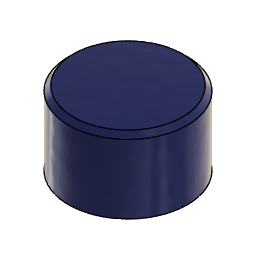
MacropadV2.0 v51 (Autodesk Fusion 360 archive; units mm, degrees)
design "knob"
Autodesk Fusion 360 part; units mm, degrees
sketch "Sketch1" plane through (0, 0, 0) normal (0, 0, 1) x (1, 0, 0)
  circle A0 centre (0, 0) radius 12.5
  circle A1 centre (0, 0) radius 3
  line L0 (0, 2.5) -> (-1.6583, 2.5)
  line L1 (0, 2.5) -> (1.6583, 2.5)
  circle A2 centre (0, 0) radius 11
  dimension "d1" = 25
  dimension "d2" = 6
  dimension "d10" = 22
  constraint coincident A0.centre A1.centre
  constraint concentric A0 A1
  constraint coincident A1 L0.end
  constraint coincident A1 L1.end
  constraint concentric A1 A2
  measures "d1" diameter of A0
  measures "d2" diameter of A1
  measures "d10" diameter of A2
extrude "Extrude1" add sketch "Sketch1" along normal blind 15 contours A0 | A1 L0 L1 | A2 picked at (-0.1459, 2.8226)
sketch "Sketch2" plane through (0, 0, 15) normal (0, 0, 1) x (-1, 0, 0)
  arc A0 (1.6583, -2.5) -> (-1.6583, -2.5) centre (0, 0) ccw
  line L0 (1.6583, -2.5) -> (-1.6583, -2.5)
  circle A1 centre (0, 0) radius 12.5
  line L1 (1.6583, -2.5) -> (-1.6583, -2.5)
  arc A2 (1.6583, -2.5) -> (-1.6583, -2.5) centre (0, 0) ccw
  dimension "d6" = 0
  measures "d6" distance of L0
extrude "Extrude2" add sketch "Sketch2" against normal blind 5 contours A0 L0 L1 A2
extrude "Extrude3" cut sketch "Sketch1" along normal blind 2.5 contours A1 L0 L1 | A2 picked at (-0.1459, 2.8226)
chamfer "Chamfer1" distance 1 angle 45 1 edges at (-11.6541, -4.5202, 15)
move_face "OffsetFaces1" offset 0.5 1 faces at (11.9125, -1.1675, 0)
delete_face "DeleteFace1" 1 faces at (-0.5528, 2.5, 7.5)
move_face "OffsetFaces2" offset -3.9 1 faces at (-1.0105, -0.7891, 10)

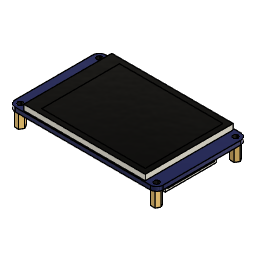
design "2inchLCD_Display"
Autodesk Fusion 360 part; units mm, degrees
sketch "Sketch1" plane through (0, 0, 0) normal (0, 0, 1) x (1, 0, 0)
  line L0 (2.5, 0) -> (55.5, 0)
  line L1 (58, 2.5) -> (58, 33)
  line L2 (55.5, 35.5) -> (2.5, 35.5)
  line L3 (0, 33) -> (0, 2.5)
  line L4 (0, 0) -> (2.25, 0) construction
  line L5 (2.25, 0) -> (2.25, 2.25) construction
  line L6 (2.25, 2.25) -> (0, 2.25) construction
  line L7 (0, 2.25) -> (0, 0) construction
  circle A0 centre (2.25, 2.25) radius 1
  line L8 (0, 35.5) -> (2.25, 35.5) construction
  line L9 (2.25, 35.5) -> (2.25, 33.25) construction
  line L10 (2.25, 33.25) -> (0, 33.25) construction
  line L11 (0, 33.25) -> (0, 35.5) construction
  circle A1 centre (2.25, 33.25) radius 1
  line L12 (58, 35.5) -> (55.75, 35.5) construction
  line L13 (55.75, 35.5) -> (55.75, 33.25) construction
  line L14 (55.75, 33.25) -> (58, 33.25) construction
  line L15 (58, 33.25) -> (58, 35.5) construction
  circle A2 centre (55.75, 33.25) radius 1
  line L16 (58, 0) -> (55.75, 0) construction
  line L17 (55.75, 0) -> (55.75, 2.25) construction
  line L18 (55.75, 2.25) -> (58, 2.25) construction
  line L19 (58, 2.25) -> (58, 0) construction
  circle A3 centre (55.75, 2.25) radius 1
  arc A4 (58, 33) -> (55.5, 35.5) centre (55.5, 33) ccw
  arc A5 (55.5, 0) -> (58, 2.5) centre (55.5, 2.5) ccw
  arc A6 (0, 2.5) -> (2.5, 0) centre (2.5, 2.5) ccw
  arc A7 (2.5, 35.5) -> (0, 33) centre (2.5, 33) ccw
  line L20 (53, 35) -> (53, 0.5)
  line L21 (53, 35) -> (5.4, 35)
  line L22 (53, 0.5) -> (5.4, 0.5)
  line L23 (5.4, 35) -> (5.4, 0.5)
  line L24 (53, 35) -> (51, 35) construction
  line L25 (51, 35) -> (51, 33) construction
  line L26 (51, 33) -> (53, 33) construction
  line L27 (53, 33) -> (53, 35) construction
  line L28 (5.4, 0.5) -> (10.4, 0.5) construction
  line L29 (10.4, 0.5) -> (10.4, 2.5) construction
  line L30 (10.4, 2.5) -> (5.4, 2.5) construction
  line L31 (5.4, 2.5) -> (5.4, 0.5) construction
  line L32 (51, 33) -> (10.4, 33)
  line L33 (10.4, 33) -> (10.4, 2.5)
  line L34 (10.4, 2.5) -> (51, 2.5)
  line L35 (51, 2.5) -> (51, 33)
  dimension "d1" = 58
  dimension "d2" = 35.5
  dimension "d17" = 2.25
  dimension "d18" = 2.25
  dimension "d19" = 2
  dimension "d20" = 2.25
  dimension "d21" = 2.25
  dimension "d22" = 2
  dimension "d23" = 2.25
  dimension "d24" = 2.25
  dimension "d25" = 2
  dimension "d26" = 2.25
  dimension "d27" = 2.25
  dimension "d28" = 2
  dimension "d29" = 2.5
  dimension "d32" = 34.5
  dimension "d33" = 47.6
  dimension "d34" = 47.6
  dimension "d36" = 2
  dimension "d37" = 2
  dimension "d38" = 5
  dimension "d39" = 2
  constraint horizontal L0
  constraint vertical L1
  constraint horizontal L2
  constraint vertical L3
  constraint coincident L4.start L7.end
  constraint horizontal L4
  constraint vertical L5
  constraint horizontal L6
  constraint vertical L7
  constraint coincident L5.end L6.start
  constraint horizontal L8
  constraint vertical L9
  constraint horizontal L10
  constraint vertical L11
  constraint coincident L9.end L10.start
  constraint horizontal L12
  constraint vertical L13
  constraint horizontal L14
  constraint vertical L15
  constraint coincident L13.end L14.start
  constraint horizontal L16
  constraint vertical L17
  constraint horizontal L18
  constraint vertical L19
  constraint coincident L17.end L18.start
  constraint coincident L12.start L1
  constraint coincident L12.start L2
  constraint tangent L1 A4
  constraint tangent L2 A4
  constraint coincident L16.start L0
  constraint coincident L16.start L1
  constraint tangent L0 A5
  constraint tangent L1 A5
  constraint equal A4 A5
  constraint coincident L4.start L0
  constraint coincident L4.start L3
  constraint tangent L0 A6
  constraint tangent L3 A6
  constraint equal A4 A6
  constraint coincident L8.start L3
  constraint coincident L8.start L2
  constraint tangent L3 A7
  constraint tangent L2 A7
  constraint equal A4 A7
  constraint perpendicular L2 L20
  constraint perpendicular L20 L21
  constraint perpendicular L20 L22
  constraint horizontal L24
  constraint vertical L25
  constraint horizontal L26
  constraint vertical L27
  constraint horizontal L28
  constraint vertical L29
  constraint horizontal L30
  constraint vertical L31
  constraint horizontal L32
  constraint vertical L33
  constraint horizontal L34
  constraint vertical L35
  measures "d1" distance of L4.start L16.start
  measures "d2" distance of L4.start L8.start
  measures "d17" distance of L4.start L4.end
  measures "d18" distance of L4.start L6.end
  measures "d19" diameter of A0
  measures "d20" distance of L8.start L8.end
  measures "d21" distance of L8.start L10.end
  measures "d22" diameter of A1
  measures "d23" distance of L12.start L12.end
  measures "d24" distance of L12.start L14.end
  measures "d25" diameter of A2
  measures "d26" distance of L16.start L16.end
  measures "d27" distance of L16.start L18.end
  measures "d28" diameter of A3
  measures "d29" radius of A4
  measures "d32" distance of L20.start L20.end
  measures "d33" distance of L20.start L21.end
  measures "d34" distance of L20.end L22.end
  measures "d36" distance of L20.start L24.end
  measures "d37" distance of L20.start L26.end
  measures "d38" distance of L22.end L28.end
  measures "d39" distance of L22.end L30.end
extrude "Extrude1" add sketch "Sketch1" against normal blind 1.6 contours L0 L1 L2 L3 A4 A5 A6 A7 | L20 L21 L22 L23 | L32 L33 L34 L35 makes body 1
extrude "Extrude2" add sketch "Sketch1" along normal blind 2.2 contours L20 L21 L22 L23 bodies 1
extrude "Extrude3" add sketch "Sketch1" along normal blind 2.19 contours L32 L33 L34 L35 bodies 1
sketch "Sketch2" plane through (0, 0, -1.6) normal (0, 0, -1) x (1, 0, 0)
  circle A0 centre (2.25, -2.25) radius 1
  circle A1 centre (55.75, -2.25) radius 1
  circle A2 centre (2.25, -33.25) radius 1
  circle A3 centre (55.75, -33.25) radius 1
  arc A4 (0, -33) -> (2.5, -35.5) centre (2.5, -33) ccw
  line L0 (2.5, -35.5) -> (55.5, -35.5)
  arc A5 (55.5, -35.5) -> (58, -33) centre (55.5, -33) ccw
  line L1 (58, -33) -> (58, -2.5)
  arc A6 (58, -2.5) -> (55.5, 0) centre (55.5, -2.5) ccw
  line L2 (55.5, 0) -> (2.5, 0)
  arc A7 (2.5, 0) -> (0, -2.5) centre (2.5, -2.5) ccw
  line L3 (0, -2.5) -> (0, -33)
  line L4 (53.6, -27.75) -> (53.6, -7.75)
  line L5 (53.6, -27.75) -> (47.6, -27.75)
  line L6 (47.6, -27.75) -> (47.6, -7.75)
  line L7 (47.6, -7.75) -> (53.6, -7.75)
  line L8 (47.6, -27.75) -> (46, -27.75)
  line L9 (46, -27.75) -> (46, -27.15)
  line L10 (46, -27.15) -> (47.6, -27.15)
  line L11 (47.6, -27.15) -> (47.6, -27.75)
  line L12 (47.6, -7.75) -> (46, -7.75)
  line L13 (46, -7.75) -> (46, -8.35)
  line L14 (46, -8.35) -> (47.6, -8.35)
  line L15 (47.6, -8.35) -> (47.6, -7.75)
  dimension "d48" = 20
  dimension "d49" = 6
  dimension "d50" = 20
  dimension "d51" = 1.6
  dimension "d52" = 0.6
  dimension "d53" = 1.6
  dimension "d54" = 0.6
  constraint horizontal L5
  constraint vertical L6
  constraint horizontal L7
  constraint horizontal L8
  constraint vertical L9
  constraint horizontal L10
  constraint vertical L11
  constraint horizontal L12
  constraint vertical L13
  constraint horizontal L14
  constraint vertical L15
  measures "d48" distance of L4.start L4.end
  measures "d49" distance of L4.start L5.end
  measures "d50" distance of L4.start L4.end
  measures "d51" distance of L5.end L8.end
  measures "d52" distance of L5.end L10.end
  measures "d53" distance of L6.end L12.end
  measures "d54" distance of L6.end L14.end
extrude "Extrude4" add sketch "Sketch2" along normal blind 5.6 contours L4 L5 L6 L7 L11 L15 bodies 1
extrude "Extrude5" add sketch "Sketch2" along normal blind 2.5 contours L6 L8 L9 L10 L11 | L6 L12 L13 L14 L15 bodies 1
chamfer "Chamfer1" distance 1.6 angle 45 2 edges at (47.6, 27.45, -4.1) (47.6, 8.05, -4.1) on bodies 1
sketch "Sketch3" plane through (53.6, 0, 0) normal (1, 0, 0) x (0, 1, 0)
  line L0 (27.75, -1.6) -> (7.75, -1.6)
  line L1 (7.75, -1.6) -> (7.75, -7.2)
  line L2 (7.75, -7.2) -> (27.75, -7.2)
  line L3 (27.75, -7.2) -> (27.75, -1.6)
  line L4 (26.95, -2.4) -> (8.55, -2.4)
  line L5 (8.55, -2.4) -> (8.55, -6.4)
  line L6 (8.55, -6.4) -> (26.95, -6.4)
  line L7 (26.95, -6.4) -> (26.95, -2.4)
  line L8 (26.95, -4.4) -> (25.9, -4.4)
  line L9 (26.2, -4.1) -> (25.6, -4.1)
  line L10 (25.6, -4.1) -> (25.6, -4.7)
  line L11 (25.6, -4.7) -> (26.2, -4.7)
  line L12 (26.2, -4.7) -> (26.2, -4.1)
  line L13 (23.3143, -4.7) -> (23.9143, -4.7)
  line L14 (23.9143, -4.7) -> (23.9143, -4.1)
  line L15 (23.9143, -4.1) -> (23.3143, -4.1)
  line L16 (23.3143, -4.1) -> (23.3143, -4.7)
  line L17 (21.0286, -4.7) -> (21.6286, -4.7)
  line L18 (21.6286, -4.7) -> (21.6286, -4.1)
  line L19 (21.6286, -4.1) -> (21.0286, -4.1)
  line L20 (21.0286, -4.1) -> (21.0286, -4.7)
  line L21 (18.7429, -4.7) -> (19.3429, -4.7)
  line L22 (19.3429, -4.7) -> (19.3429, -4.1)
  line L23 (19.3429, -4.1) -> (18.7429, -4.1)
  line L24 (18.7429, -4.1) -> (18.7429, -4.7)
  line L25 (16.4571, -4.7) -> (17.0571, -4.7)
  line L26 (17.0571, -4.7) -> (17.0571, -4.1)
  line L27 (17.0571, -4.1) -> (16.4571, -4.1)
  line L28 (16.4571, -4.1) -> (16.4571, -4.7)
  line L29 (14.1714, -4.7) -> (14.7714, -4.7)
  line L30 (14.7714, -4.7) -> (14.7714, -4.1)
  line L31 (14.7714, -4.1) -> (14.1714, -4.1)
  line L32 (14.1714, -4.1) -> (14.1714, -4.7)
  line L33 (11.8857, -4.7) -> (12.4857, -4.7)
  line L34 (12.4857, -4.7) -> (12.4857, -4.1)
  line L35 (12.4857, -4.1) -> (11.8857, -4.1)
  line L36 (11.8857, -4.1) -> (11.8857, -4.7)
  line L37 (9.6, -4.7) -> (10.2, -4.7)
  line L38 (10.2, -4.7) -> (10.2, -4.1)
  line L39 (10.2, -4.1) -> (9.6, -4.1)
  line L40 (9.6, -4.1) -> (9.6, -4.7)
  point P0 (25.9, -4.4)
  dimension "d60" = -0.8
  dimension "d61" = 1.05
  dimension "d62" = 0.6
  dimension "d63" = 0.6
  dimension "d66" = -16
  dimension "d67" = 0
  constraint midpoint L7 L8.start
  constraint perpendicular L7 L8
  constraint horizontal L9
  constraint perpendicular L9 L10
  constraint parallel L9 L11
  constraint parallel L10 L12
  constraint coincident P0 L8.end
  measures "d61" distance of L8.start P0
  measures "d62" distance of L10.end L11.end
  measures "d63" distance of L9.end L10.end
extrude "Extrude6" cut sketch "Sketch3" against normal blind 5 contours L4 L5 L6 L7 bodies 1
sketch "Sketch4" plane through (0, 0, -1.6) normal (0, 0, -1) x (1, 0, 0)
  line L0 (53.6, -27.75) -> (46, -27.75)
  line L1 (46, -27.75) -> (46, -27.15)
  line L2 (46, -27.15) -> (47.6, -27.15)
  line L3 (47.6, -27.15) -> (47.6, -8.35)
  line L4 (47.6, -8.35) -> (46, -8.35)
  line L5 (46, -8.35) -> (46, -7.75)
  line L6 (46, -7.75) -> (53.6, -7.75)
  line L7 (53.6, -7.75) -> (53.6, -27.75)
  circle A0 centre (2.25, -2.25) radius 1
  circle A1 centre (55.75, -2.25) radius 1
  circle A2 centre (2.25, -33.25) radius 1
  circle A3 centre (55.75, -33.25) radius 1
  arc A4 (0, -33) -> (2.5, -35.5) centre (2.5, -33) ccw
  line L8 (2.5, -35.5) -> (55.5, -35.5)
  arc A5 (55.5, -35.5) -> (58, -33) centre (55.5, -33) ccw
  line L9 (58, -33) -> (58, -2.5)
  arc A6 (58, -2.5) -> (55.5, 0) centre (55.5, -2.5) ccw
  line L10 (55.5, 0) -> (2.5, 0)
  arc A7 (2.5, 0) -> (0, -2.5) centre (2.5, -2.5) ccw
  line L11 (0, -2.5) -> (0, -33)
  line L12 (3.116, -3.75) -> (3.9821, -2.25)
  line L13 (3.9821, -2.25) -> (3.116, -0.75)
  line L14 (3.116, -0.75) -> (1.384, -0.75)
  line L15 (1.384, -0.75) -> (0.5179, -2.25)
  line L16 (0.5179, -2.25) -> (1.384, -3.75)
  line L17 (1.384, -3.75) -> (3.116, -3.75)
  point P0 (2.25, -2.25)
  dimension "d70" = 1.5
  constraint coincident P0 A0.centre
  measures "d70" distance of P0 L17
extrude "Extrude7" add sketch "Sketch4" along normal blind 6 separate body contours L12 L13 L14 L15 L16 L17 makes body 2
copy_body "CopyPasteBodies1" bodies 2 makes body 3
move_body "Move1" bodies 3 to x (1, 0, 0) y (0, 1, 0) z (0, 0, 1) at (0, 31, 0)
copy_body "CopyPasteBodies2" bodies 2 makes body 4
move_body "Move2" bodies 4 to x (1, 0, 0) y (0, 1, 0) z (0, 0, 1) at (53.5, 0, 0)
copy_body "CopyPasteBodies3" bodies 4 makes body 5
move_body "Move3" bodies 5 to x (1, 0, 0) y (0, 1, 0) z (0, 0, 1) at (0, 31, 0)

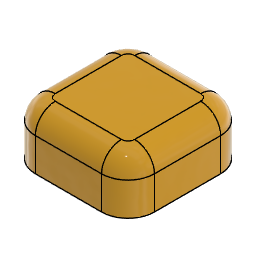
design "keycap"
Autodesk Fusion 360 part; units mm, degrees
sketch "Sketch1" plane through (0, 0, 0) normal (0, 0, 1) x (1, 0, 0)
  line L0 (0, 0) -> (18, 0)
  line L1 (18, 0) -> (18, 18)
  line L2 (18, 18) -> (0, 18)
  line L3 (0, 18) -> (0, 0)
  circle A0 centre (9, 9) radius 2.5
  line L4 (5, 1) -> (13, 1)
  line L5 (17, 5) -> (17, 13)
  line L6 (13, 17) -> (5, 17)
  line L7 (1, 13) -> (1, 5)
  arc A1 (17, 13) -> (13, 17) centre (13, 13) ccw
  arc A2 (5, 17) -> (1, 13) centre (5, 13) ccw
  arc A3 (1, 5) -> (5, 1) centre (5, 5) ccw
  arc A4 (13, 1) -> (17, 5) centre (13, 5) ccw
  dimension "d1" = 18
  dimension "d2" = 18
  dimension "d3" = 5
  dimension "d11" = 4
  constraint horizontal L0
  constraint vertical L1
  constraint horizontal L2
  constraint vertical L3
  constraint coincident L0.start L3.end
  constraint tangent L5 A1
  constraint tangent L6 A1
  constraint tangent L6 A2
  constraint tangent L7 A2
  constraint equal A1 A2
  constraint tangent L4 A3
  constraint tangent L7 A3
  constraint equal A1 A3
  constraint tangent L4 A4
  constraint tangent L5 A4
  constraint equal A1 A4
  measures "d1" distance of L0.start L0.end
  measures "d2" distance of L0.start L2.end
  measures "d3" diameter of A0
  measures "d11" radius of A1
extrude "Extrude1" add sketch "Sketch1" along normal blind 8 contours L0 L1 L2 L3 | A0 | L4 L5 L6 L7 A1 A2 A3 A4
fillet "Fillet1" radius 3 4 edges at (9, 0, 8) (0, 9, 8) (9, 18, 8) (18, 9, 8)
fillet "Fillet2" radius 4 8 edges at (18, 0, 2.5) (17.1213, 0.8787, 7.1213) (0, 0, 2.5) (0.8787, 0.8787, 7.1213) (0.8787, 17.1213, 7.1213) (0, 18, 2.5) (17.1213, 17.1213, 7.1213) (18, 18, 2.5)
extrude "Extrude2" cut sketch "Sketch1" along normal blind 4 contours L4 L5 L6 L7 A1 A2 A3 A4
sketch "Sketch2" plane through (0, 0, 0) normal (0, 0, -1) x (1, 0, 0)
  circle A0 centre (9, -9) radius 2.5
  line L0 (9.65, -7) -> (8.35, -7)
  line L1 (8.35, -7) -> (8.35, -11)
  line L2 (8.35, -11) -> (9.65, -11)
  line L3 (9.65, -11) -> (9.65, -7)
  line L4 (9.65, -7) -> (8.35, -11) construction
  line L5 (8.35, -7) -> (9.65, -11) construction
  line L6 (11, -8.35) -> (7, -8.35)
  line L7 (7, -8.35) -> (7, -9.65)
  line L8 (7, -9.65) -> (11, -9.65)
  line L9 (11, -9.65) -> (11, -8.35)
  line L10 (11, -8.35) -> (7, -9.65) construction
  line L11 (7, -8.35) -> (11, -9.65) construction
  point P0 (9, -9)
  point P1 (9, -9)
  dimension "d14" = 1.3
  dimension "d15" = 4
  dimension "d16" = 4
  dimension "d17" = 1.3
  constraint horizontal L0
  constraint perpendicular L0 L1
  constraint parallel L0 L2
  constraint parallel L1 L3
  constraint coincident L4 P1
  constraint coincident L5 P1
  constraint coincident P0 A0.centre
  constraint horizontal L6
  constraint perpendicular L6 L7
  constraint parallel L6 L8
  constraint parallel L7 L9
  constraint coincident L10 P1
  constraint coincident L11 P1
  constraint coincident P1 P0
  measures "d14" distance of L1.end L2.end
  measures "d15" distance of L0.end L1.end
  measures "d16" distance of L7.end L8.end
  measures "d17" distance of L6.end L7.end
extrude "Extrude3" cut sketch "Sketch2" against normal blind 3 contours L0 L1 L3 L6 | L3 L6 L8 L9 | L1 L3 L6 L8 | L1 L6 L7 L8 | L1 L2 L3 L8
